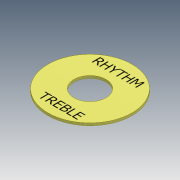
# Autodesk Inventor part: RHYTHM & TREBLE 2
Saved by Autodesk Inventor 2016 (Build 200138000, 138)
## iProperties
Created: 2018-11-13
Part Number: RHYTHM & TREBLE 2
Material: Genérico
Document SubType Name: Modeling
Designer: thiag
Density: 1 g/cm^3
Appearance: Yellow(1)
Author: thiag
Autodesk Inventor part; units mm, degrees
ref_plane "YZ Plane" through (0, 0, 0) normal (1, 0, 0) x (0, 1, 0)
ref_plane "XZ Plane" through (0, 0, 0) normal (0, 1, 0) x (-1, 0, 0)
ref_plane "XY Plane" through (0, 0, 0) normal (0, 0, 1) x (1, 0, 0)
sketch "Esboço1" plane through (0, 0, 0) normal (0, 0, 1) x (1, 0, 0)
  circle A0 centre (0, 0) radius 17
  circle A1 centre (0, 0) radius 6.5
  constraints: 2 centre point, 2 coincident
extrude "Extrusão1" add sketch "Esboço1" along normal blind 1
sketch "Esboço2" plane through (0, 0, 1) normal (0, 0, 1) x (1, 0, 0)
  line L0 (-9.3517, 13.1144) -> (9.4303, 13.1144) construction
  line L1 (9.4303, 13.1144) -> (9.4303, 9.6144) construction
  line L2 (9.4303, 9.6144) -> (-9.3517, 9.6144) construction
  line L3 (-9.3517, 9.6144) -> (-9.3517, 13.1144) construction
  line L4 (-7.9636, -10.0458) -> (8.4643, -10.0458) construction
  line L5 (8.4643, -10.0458) -> (8.4643, -13.5458) construction
  line L6 (8.4643, -13.5458) -> (-7.9636, -13.5458) construction
  line L7 (-7.9636, -13.5458) -> (-7.9636, -10.0458) construction
  constraints: 4 other
